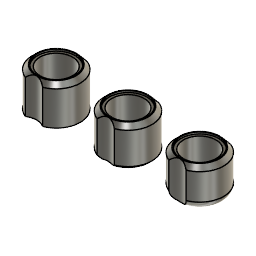
bradan_lane_coin_polishing_tool_parametric (Autodesk Fusion 360 design; units mm, degrees)
Autodesk Fusion 360 part; units mm, degrees
sketch "Main Geometry" plane through (0, 0, 0) normal (0, 0, 1) x (1, 0, 0)
  circle A0 centre (0, 0) radius 19.125
  circle A1 centre (0, 0) radius 22.125
  circle A2 centre (0, 0) radius 28.125
  circle A3 centre (0, -41.125) radius 18
  circle A4 centre (84.375, -41.125) radius 18
  circle A5 centre (84.375, 0) radius 19.125
  circle A6 centre (84.375, 0) radius 22.125
  circle A7 centre (84.375, 0) radius 28.125
  circle A8 centre (168.75, -41.125) radius 18
  circle A9 centre (168.75, 0) radius 19.125
  circle A10 centre (168.75, 0) radius 22.125
  circle A11 centre (168.75, 0) radius 28.125
  line L0 (-10, 0) -> (10, 0) construction
  circle A12 centre (0, 41.125) radius 18
  circle A13 centre (84.375, 41.125) radius 18
  circle A14 centre (168.75, 41.125) radius 18
  point P0 (84.375, 0)
  point P1 (168.75, 0)
  dimension "d21" = 38.25
  dimension "d22" = 44.25
  dimension "d23" = 56.25
  dimension "d31" = 36
  dimension "d32" = 41.125
  dimension "d37" = 84.375
  dimension "d38" = 0
  constraint coincident A0.centre A1.centre
  constraint horizontal L0
  constraint symmetric A3 L0 A12
  measures "d21" diameter of A0
  measures "d22" diameter of A1
  measures "d23" diameter of A2
  measures "d31" diameter of A3
  measures "d32" distance of A0.centre A3.centre
extrude "Extrude1" add sketch "Main Geometry" along normal blind 45 contours A1 | A2 A3 A12 | A2 A12 | A2 A3 | A4 A7 | A4 A7 A13 | A7 A13 | A6 | A8 A11 | A8 A11 A14 | A11 A14 | A10 picked at (0, 26.4075) picked at (0, -26.4075) picked at (84.375, -26.4075) picked at (84.375, 26.4075) picked at (168.75, -26.4075) picked at (168.75, 26.4075) makes body 1 at (27.9852, -2.8003, 15) makes body 2 at (112.3602, -2.8003, 15) makes body 3 at (196.7352, -2.8003, 15)
sketch "Edge Treatment" plane through (0, 0, 0) normal (0, 1, 0) x (1, 0, 0)
  line L0 (0, 0) -> (0, -45) construction
  line L1 (-28.125, -45) -> (-28.125, -40)
  line L2 (-28.125, -45) -> (-23.125, -45)
  line L3 (-23.125, -45) -> (-28.125, -40)
  line L4 (0, 0) -> (-28.125, 0) construction
  line L5 (84.375, 0) -> (56.25, 0) construction
  line L6 (61.25, -45) -> (56.25, -40)
  line L7 (84.375, 0) -> (84.375, -45) construction
  line L8 (56.25, -45) -> (61.25, -45)
  line L9 (56.25, -45) -> (56.25, -40)
  line L10 (168.75, 0) -> (140.625, 0) construction
  line L11 (145.625, -45) -> (140.625, -40)
  line L12 (168.75, 0) -> (168.75, -45) construction
  line L13 (140.625, -45) -> (145.625, -45)
  line L14 (140.625, -45) -> (140.625, -40)
  point P0 (84.375, 0)
  point P1 (168.75, 0)
  dimension "d45" = 5
  dimension "d46" = 5
  dimension "d47" = 28.125
  dimension "d48" = 28.125
  dimension "d49" = 45
  dimension "d53" = 84.375
  dimension "d54" = 0
  constraint coincident L0.start L4.start
  constraint vertical L0
  constraint vertical L1
  constraint perpendicular L1 L2
  constraint perpendicular L0 L4
  measures "d45" distance of L1.start L1.end
  measures "d46" distance of L1.start L2.end
  measures "d47" distance of L0 L1
  measures "d48" distance of L0.start L4.end
  measures "d49" distance of L2 L4
revolve "Revolve1" cut sketch "Edge Treatment" angle 360 about axis through (0, 0, 0) along (0, 0, 1) contours L1 L2 L3 bodies 1
extrude "Extrude2" cut sketch "Main Geometry" against normal blind 2 from surface at 45 contours A1 | A6 | A10 bodies 1 2 3
chamfer "Chamfer3" distance 3 angle 45 1 edges at (58.1533, -10.1704, 0) measured on face at (112.3602, -2.8003, 15) on bodies 2
fillet "Fillet1" radius 9 1 edges at (142.5283, -10.1704, 0) on bodies 3
extrude "Extrude3" cut sketch "Main Geometry" along normal blind 45 contours A2 A12 | A2 A3 | A4 A7 | A7 A13 | A8 A11 | A11 A14 picked at (0, 26.4075) picked at (0, -26.4075) picked at (84.375, -26.4075) picked at (84.375, 26.4075) picked at (168.75, -26.4075) picked at (168.75, 26.4075) bodies 1 2 3
revolve "Revolve2" cut sketch "Edge Treatment" angle 360 about axis through (84.375, 0, 0) along (0, 0, 1) contours L6 L8 L9 bodies 2
revolve "Revolve3" cut sketch "Edge Treatment" angle 360 about axis through (168.75, 0, 0) along (0, 0, 1) contours L11 L13 L14 bodies 3
equation "overall_height = 45 mm"
equation "coin_recess_depth = 2 mm"
equation "coin_recess_dia = coin_dia + coin_pocket_clearance"
equation "inner_dia_offset = 6 mm"
equation "top_outer_dia_offset = 2 mm"
equation "chamfer_height = 5 mm"
equation "chamfer_angle = 45 deg"
equation "bottom_fillet_radius = body_outer_radius - ( coin_recess_dia - inner_dia_offset ) / 2"
equation "bottom_chamfer_height = 3 mm"
equation "bottom_chamfer_angle = 45 deg"
equation "finger_cut_dia = 36 mm"
equation "inner_dia = coin_recess_dia - inner_dia_offset"
equation "top_outer_dia = coin_recess_dia + top_outer_dia_offset"
equation "top_chamfer_radial_change = chamfer_height / tan(chamfer_angle)"
equation "body_outer_dia = top_outer_dia + top_chamfer_radial_change * 2"
equation "bottom_chamfer_radial_change = bottom_chamfer_height / tan(bottom_chamfer_angle)"
equation "body_outer_radius = body_outer_dia / 2"
equation "top_outer_radius = top_outer_dia / 2"
equation "finger_cut_radius = finger_cut_dia / 2"
equation "finger_cut_offset = top_outer_radius + finger_cut_radius"
equation "d21 = inner_dia"
equation "d22 = coin_recess_dia"
equation "d23 = body_outer_dia"
equation "d24 = overall_height"
equation "d26 = overall_height"
equation "d27 = -coin_recess_depth"
equation "d31 = finger_cut_dia"
equation "d32 = finger_cut_offset"
equation "d33 = overall_height"
equation "d37 = body_outer_dia * 1.5"
equation "d41 = bottom_chamfer_height"
equation "d42 = bottom_chamfer_angle"
equation "d44 = bottom_fillet_radius"
equation "d45 = chamfer_height"
equation "d46 = top_chamfer_radial_change"
equation "d47 = body_outer_radius"
equation "d48 = body_outer_radius"
equation "d49 = overall_height"
equation "d53 = body_outer_dia * 1.5"
equation "coin_dia = 44 mm"
equation "coin_pocket_clearance = 0.25 mm"
named bodies: "Flat Model", "Chamfer Model", "Fillet Model"
